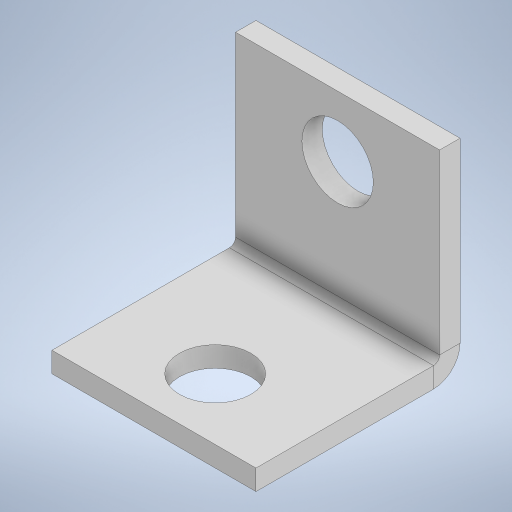
# Autodesk Inventor part: joint
Saved by Autodesk Inventor 2023 (Build 270158000, 158)
## iProperties
Created: 2023-04-07
Part Number: joint
Material: Generic
Document SubType Name: Sheet Metal
Designer: 310611102
Density: 1 g/cm^3
Sheet Metal Rule: Default_mm
Appearance: Default
Author: 310611102
Autodesk Inventor part; units mm, degrees
ref_plane "YZ Plane" through (0, 0, 0) normal (1, 0, 0) x (0, 1, 0)
ref_plane "XZ Plane" through (0, 0, 0) normal (0, 1, 0) x (-1, 0, 0)
ref_plane "XY Plane" through (0, 0, 0) normal (0, 0, 1) x (1, 0, 0)
sketch "Sketch1" plane through (0, 0, 0) normal (0, 0, 1) x (1, 0, 0)
  line L0 (0, 0) -> (10, 0)
  line L1 (10, 0) -> (10, 10)
  line L2 (10, 10) -> (0, 10)
  line L3 (0, 10) -> (0, 0)
  dimension "d0" = 10
  dimension "d1" = 10
  measures "d0" distance of L1.end L2.end
  measures "d1" distance of L0.end L1.end
extrude "Plate1" add sketch "Sketch1" along normal blind 1
sketch "Sketch2" plane through (10, 1, 0) normal (0, -1, 0) x (1, 0, 0)
  line L0 (-10, 0) -> (0, 0)
  line L1 (0, 0) -> (0, 10)
  line L2 (0, 10) -> (-10, 10)
  line L3 (-10, 10) -> (-10, 0)
  constraints: 6 end point, 1 horizontal, 1 perpendicular, 1 vertical
edge flange "Flange1" height 10 angle 90 thickness 1 bend radius 0.3 thickness toward (0, -1, 0) relief tear relief width 1 relief depth 0.5 edges at (5, 0, 1) wall of the first edge with corners at (0, 1, 0) (10, 1, 0) (10, 1, 10) (0, 1, 10)
bend "Bend1"
corner "Corner1"
sketch "Sketch3" plane through (0, 0, 0) normal (0, 0, -1) x (-1, 0, 0)
  circle A0 centre (-5, 7) radius 1.75
  line L0 (-10, 10) -> (0, 10) projected
  line L1 (-10, 1) -> (0, 1) projected
  point P0 (0, 0)
  point P1 (-5, 10)
  dimension "d13" = 3.5
  dimension "d14" = 6
  constraints: 1 centre point, 1 midpoint, 1 vertical alignment
  measures "d13" diameter of A0
  measures "d14" distance from line of L1 A0.centre
extrude "Extrusion1" cut sketch "Sketch3" against normal blind 10
sketch "Sketch4" plane through (0, 0, 10) normal (0, -1, 0) x (1, 0, 0)
  circle A0 centre (5, -3) radius 1.75
  line L0 (0, -9) -> (10, -9) projected
  line L1 (0, 0) -> (10, 0) projected
  point P0 (0, -10)
  point P1 (5, 0)
  dimension "d17" = 3.5
  dimension "d18" = 6
  constraints: 1 centre point, 1 midpoint, 1 vertical alignment
  measures "d17" diameter of A0
  measures "d18" distance from line of L0 A0.centre
extrude "Extrusion2" cut sketch "Sketch4" against normal blind 10
equation "\"d2\" = 厚度"
equation "\"d3\" = 折彎離隙寬度"
equation "\"d4\" = 折彎離隙深度"
equation "\"d5\" = 最小剩餘"
equation "\"d6\" = 轉移半徑"
equation "\"d10\" = 轉角離隙大小"
equation "\"d11\" = 間隙大小"
equation "\"d12\" = Jacobi半徑大小"
equation "\"折彎半徑\" = 厚度"
equation "\"折彎離隙寬度\" = 厚度"
equation "\"折彎離隙深度\" = 0.5 * 厚度"
equation "\"轉角離隙大小\" = 4 * 厚度"
equation "\"最小剩餘\" = 2 * 厚度"
equation "\"轉移半徑\" = 折彎半徑"
equation "\"Jacobi半徑大小\" = 折彎半徑"
equation "\"間隙大小\" = 厚度"
equation "\"厚度\" = 1"
body "Solid1"
